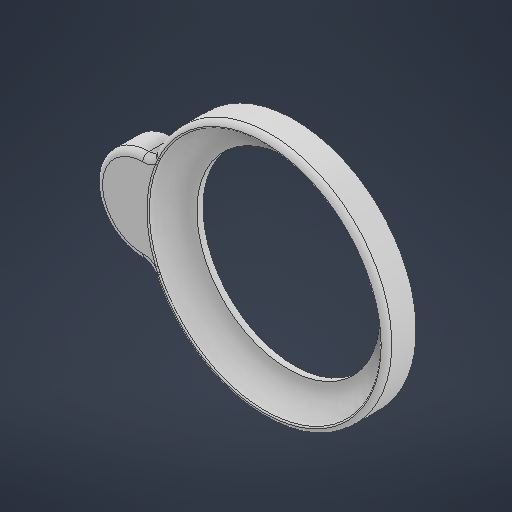
# Autodesk Inventor part: Shottfiller Adapter
Saved by Autodesk Inventor 2026.2 (Build 302298000, 298)
## iProperties
Created: 2025-12-11
Part Number: Shottfiller Adapter
Material: Generic
Document SubType Name: Modeling
Designer: bubim
Density: 1 g/cm^3
Appearance: Default
Author: bubim
Autodesk Inventor part; units mm, degrees
ref_plane "YZ Plane" through (0, 0, 0) normal (1, 0, 0) x (0, 1, 0)
ref_plane "XZ Plane" through (0, 0, 0) normal (0, 1, 0) x (-1, 0, 0)
ref_plane "XY Plane" through (0, 0, 0) normal (0, 0, 1) x (1, 0, 0)
sketch "Sketch1" plane through (0, 0, 0) normal (0, 0, 1) x (1, 0, 0)
  arc A0 (-18.012543, -8.634172) -> (-18.012543, 8.634172) centre (0, 0) ccw
  arc A1 (-19.849514, 7.49895) -> (-19.849514, -7.49895) centre (-19.975, 0) ccw
  arc A2 (-19.849514, 7.49895) -> (-18.012543, 8.634172) centre (-19.816051, 9.49867) ccw
  arc A3 (-18.012543, -8.634172) -> (-19.849514, -7.49895) centre (-19.816051, -9.49867) ccw
  circle A4 centre (0, 0) radius 15
  dimension "d0" = 39.95
  dimension "d1" = 15
  dimension "d2" = 2
  dimension "d3" = 30
  constraints: 9 point on circle, 5 centre point, 4 tangent, 2 coincident, 1 equal radius, 1 horizontal alignment
  measures "d0" diameter of A0
  measures "d1" diameter of A1
  measures "d2" radius of A2
  measures "d3" diameter of A4
extrude "Extrusion1" add sketch "Sketch1" along normal mid plane 5
fillet "Fillet1" radius 4 1 edges at (-15, 0, 2.5) inverted yes
fillet "Fillet4" radius 1 4 edges at (-18.7646, 7.7973, 2.5) (-27.475, 0, 2.5) (-18.7646, -7.7973, 2.5) (19.975, 0, 2.5) curvature continuous yes
fillet "Fillet5" radius 0.2 7 edges at (4.2111, 18.5275, 2.5) (4.2111, -18.5274, 2.5) (-17.2043, -8.0631, 2.5) (-17.2797, -7.9001, 2.5) (-19, 0, 2.5) (-17.2797, 7.9001, 2.5) (-17.2043, 8.0631, 2.5)
body "Solid1"
